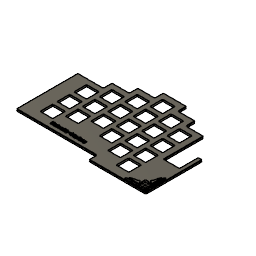
right_top (Autodesk Fusion 360 design; units mm, degrees)
part number: 2026-06-20-00-17-14-942
Autodesk Fusion 360 part; units mm, degrees
(part 1 of 2)
sketch "Sketch1" plane through (0, 0, 0) normal (0, 0, 1) x (1, 0, 0)
  line L0 (0.7819, 35.4718) -> (13.7819, 35.4718)
  line L1 (0.7819, 21.4718) -> (13.7819, 21.4718)
  line L2 (0.2819, 34.9718) -> (0.2819, 21.9718)
  line L3 (14.2819, 34.9718) -> (14.2819, 21.9718)
  arc A0 (0.7819, 35.4718) -> (0.2819, 34.9718) centre (0.7819, 34.9718) ccw
  arc A1 (14.2819, 34.9718) -> (13.7819, 35.4718) centre (13.7819, 34.9718) ccw
  arc A2 (0.2819, 21.9718) -> (0.7819, 21.4718) centre (0.7819, 21.9718) ccw
  arc A3 (13.7819, 21.4718) -> (14.2819, 21.9718) centre (13.7819, 21.9718) ccw
  line L4 (-18.2681, 25.9468) -> (-5.2681, 25.9468)
  line L5 (-18.2681, 11.9468) -> (-5.2681, 11.9468)
  line L6 (-18.7681, 25.4468) -> (-18.7681, 12.4468)
  line L7 (-4.7681, 25.4468) -> (-4.7681, 12.4468)
  arc A4 (-18.2681, 25.9468) -> (-18.7681, 25.4468) centre (-18.2681, 25.4468) ccw
  arc A5 (-4.7681, 25.4468) -> (-5.2681, 25.9468) centre (-5.2681, 25.4468) ccw
  arc A6 (-18.7681, 12.4468) -> (-18.2681, 11.9468) centre (-18.2681, 12.4468) ccw
  arc A7 (-5.2681, 11.9468) -> (-4.7681, 12.4468) centre (-5.2681, 12.4468) ccw
  line L8 (19.8319, 25.9468) -> (32.8319, 25.9468)
  line L9 (19.8319, 11.9468) -> (32.8319, 11.9468)
  line L10 (19.3319, 25.4468) -> (19.3319, 12.4468)
  line L11 (33.3319, 25.4468) -> (33.3319, 12.4468)
  arc A8 (19.8319, 25.9468) -> (19.3319, 25.4468) centre (19.8319, 25.4468) ccw
  arc A9 (33.3319, 25.4468) -> (32.8319, 25.9468) centre (32.8319, 25.4468) ccw
  arc A10 (19.3319, 12.4468) -> (19.8319, 11.9468) centre (19.8319, 12.4468) ccw
  arc A11 (32.8319, 11.9468) -> (33.3319, 12.4468) centre (32.8319, 12.4468) ccw
  line L12 (-37.3181, 16.4218) -> (-24.3181, 16.4218)
  line L13 (-37.3181, 2.4218) -> (-24.3181, 2.4218)
  line L14 (-37.8181, 15.9218) -> (-37.8181, 2.9218)
  line L15 (-23.8181, 15.9218) -> (-23.8181, 2.9218)
  arc A12 (-37.3181, 16.4218) -> (-37.8181, 15.9218) centre (-37.3181, 15.9218) ccw
  arc A13 (-23.8181, 15.9218) -> (-24.3181, 16.4218) centre (-24.3181, 15.9218) ccw
  arc A14 (-37.8181, 2.9218) -> (-37.3181, 2.4218) centre (-37.3181, 2.9218) ccw
  arc A15 (-24.3181, 2.4218) -> (-23.8181, 2.9218) centre (-24.3181, 2.9218) ccw
  line L16 (0.7819, 16.4218) -> (13.7819, 16.4218)
  line L17 (0.7819, 2.4218) -> (13.7819, 2.4218)
  line L18 (0.2819, 15.9218) -> (0.2819, 2.9218)
  line L19 (14.2819, 15.9218) -> (14.2819, 2.9218)
  arc A16 (0.7819, 16.4218) -> (0.2819, 15.9218) centre (0.7819, 15.9218) ccw
  arc A17 (14.2819, 15.9218) -> (13.7819, 16.4218) centre (13.7819, 15.9218) ccw
  arc A18 (0.2819, 2.9218) -> (0.7819, 2.4218) centre (0.7819, 2.9218) ccw
  arc A19 (13.7819, 2.4218) -> (14.2819, 2.9218) centre (13.7819, 2.9218) ccw
  line L20 (38.8819, 16.4218) -> (51.8819, 16.4218)
  line L21 (38.8819, 2.4218) -> (51.8819, 2.4218)
  line L22 (38.3819, 15.9218) -> (38.3819, 2.9218)
  line L23 (52.3819, 15.9218) -> (52.3819, 2.9218)
  arc A20 (38.8819, 16.4218) -> (38.3819, 15.9218) centre (38.8819, 15.9218) ccw
  arc A21 (52.3819, 15.9218) -> (51.8819, 16.4218) centre (51.8819, 15.9218) ccw
  arc A22 (38.3819, 2.9218) -> (38.8819, 2.4218) centre (38.8819, 2.9218) ccw
  arc A23 (51.8819, 2.4218) -> (52.3819, 2.9218) centre (51.8819, 2.9218) ccw
  line L24 (-56.3681, 6.8968) -> (-43.3681, 6.8968)
  line L25 (-56.3681, -7.1032) -> (-43.3681, -7.1032)
  line L26 (-56.8681, 6.3968) -> (-56.8681, -6.6032)
  line L27 (-42.8681, 6.3968) -> (-42.8681, -6.6032)
  arc A24 (-56.3681, 6.8968) -> (-56.8681, 6.3968) centre (-56.3681, 6.3968) ccw
  arc A25 (-42.8681, 6.3968) -> (-43.3681, 6.8968) centre (-43.3681, 6.3968) ccw
  arc A26 (-56.8681, -6.6032) -> (-56.3681, -7.1032) centre (-56.3681, -6.6032) ccw
  arc A27 (-43.3681, -7.1032) -> (-42.8681, -6.6032) centre (-43.3681, -6.6032) ccw
  line L28 (-18.2681, 6.8968) -> (-5.2681, 6.8968)
  line L29 (-18.2681, -7.1032) -> (-5.2681, -7.1032)
  line L30 (-18.7681, 6.3968) -> (-18.7681, -6.6032)
  line L31 (-4.7681, 6.3968) -> (-4.7681, -6.6032)
  arc A28 (-18.2681, 6.8968) -> (-18.7681, 6.3968) centre (-18.2681, 6.3968) ccw
  arc A29 (-4.7681, 6.3968) -> (-5.2681, 6.8968) centre (-5.2681, 6.3968) ccw
  arc A30 (-18.7681, -6.6032) -> (-18.2681, -7.1032) centre (-18.2681, -6.6032) ccw
  arc A31 (-5.2681, -7.1032) -> (-4.7681, -6.6032) centre (-5.2681, -6.6032) ccw
  line L32 (19.8319, 6.8968) -> (32.8319, 6.8968)
  line L33 (19.8319, -7.1032) -> (32.8319, -7.1032)
  line L34 (19.3319, 6.3968) -> (19.3319, -6.6032)
  line L35 (33.3319, 6.3968) -> (33.3319, -6.6032)
  arc A32 (19.8319, 6.8968) -> (19.3319, 6.3968) centre (19.8319, 6.3968) ccw
  arc A33 (33.3319, 6.3968) -> (32.8319, 6.8968) centre (32.8319, 6.3968) ccw
  arc A34 (19.3319, -6.6032) -> (19.8319, -7.1032) centre (19.8319, -6.6032) ccw
  arc A35 (32.8319, -7.1032) -> (33.3319, -6.6032) centre (32.8319, -6.6032) ccw
  line L36 (-37.3181, -2.6282) -> (-24.3181, -2.6282)
  line L37 (-37.3181, -16.6282) -> (-24.3181, -16.6282)
  line L38 (-37.8181, -3.1282) -> (-37.8181, -16.1282)
  line L39 (-23.8181, -3.1282) -> (-23.8181, -16.1282)
  arc A36 (-37.3181, -2.6282) -> (-37.8181, -3.1282) centre (-37.3181, -3.1282) ccw
  arc A37 (-23.8181, -3.1282) -> (-24.3181, -2.6282) centre (-24.3181, -3.1282) ccw
  arc A38 (-37.8181, -16.1282) -> (-37.3181, -16.6282) centre (-37.3181, -16.1282) ccw
  arc A39 (-24.3181, -16.6282) -> (-23.8181, -16.1282) centre (-24.3181, -16.1282) ccw
  line L40 (0.7819, -2.6282) -> (13.7819, -2.6282)
  line L41 (0.7819, -16.6282) -> (13.7819, -16.6282)
  line L42 (0.2819, -3.1282) -> (0.2819, -16.1282)
  line L43 (14.2819, -3.1282) -> (14.2819, -16.1282)
  arc A40 (0.7819, -2.6282) -> (0.2819, -3.1282) centre (0.7819, -3.1282) ccw
  arc A41 (14.2819, -3.1282) -> (13.7819, -2.6282) centre (13.7819, -3.1282) ccw
  arc A42 (0.2819, -16.1282) -> (0.7819, -16.6282) centre (0.7819, -16.1282) ccw
  arc A43 (13.7819, -16.6282) -> (14.2819, -16.1282) centre (13.7819, -16.1282) ccw
  line L44 (38.8819, -2.6282) -> (51.8819, -2.6282)
  line L45 (38.8819, -16.6282) -> (51.8819, -16.6282)
  line L46 (38.3819, -3.1282) -> (38.3819, -16.1282)
  line L47 (52.3819, -3.1282) -> (52.3819, -16.1282)
  arc A44 (38.8819, -2.6282) -> (38.3819, -3.1282) centre (38.8819, -3.1282) ccw
  arc A45 (52.3819, -3.1282) -> (51.8819, -2.6282) centre (51.8819, -3.1282) ccw
  arc A46 (38.3819, -16.1282) -> (38.8819, -16.6282) centre (38.8819, -16.1282) ccw
  arc A47 (51.8819, -16.6282) -> (52.3819, -16.1282) centre (51.8819, -16.1282) ccw
  line L48 (-56.3681, -12.1532) -> (-43.3681, -12.1532)
  line L49 (-56.3681, -26.1532) -> (-43.3681, -26.1532)
  line L50 (-56.8681, -12.6532) -> (-56.8681, -25.6532)
  line L51 (-42.8681, -12.6532) -> (-42.8681, -25.6532)
  arc A48 (-56.3681, -12.1532) -> (-56.8681, -12.6532) centre (-56.3681, -12.6532) ccw
  arc A49 (-42.8681, -12.6532) -> (-43.3681, -12.1532) centre (-43.3681, -12.6532) ccw
  arc A50 (-56.8681, -25.6532) -> (-56.3681, -26.1532) centre (-56.3681, -25.6532) ccw
  arc A51 (-43.3681, -26.1532) -> (-42.8681, -25.6532) centre (-43.3681, -25.6532) ccw
  line L52 (-18.2681, -12.1532) -> (-5.2681, -12.1532)
  line L53 (-18.2681, -26.1532) -> (-5.2681, -26.1532)
  line L54 (-18.7681, -12.6532) -> (-18.7681, -25.6532)
  line L55 (-4.7681, -12.6532) -> (-4.7681, -25.6532)
  arc A52 (-18.2681, -12.1532) -> (-18.7681, -12.6532) centre (-18.2681, -12.6532) ccw
  arc A53 (-4.7681, -12.6532) -> (-5.2681, -12.1532) centre (-5.2681, -12.6532) ccw
  arc A54 (-18.7681, -25.6532) -> (-18.2681, -26.1532) centre (-18.2681, -25.6532) ccw
  arc A55 (-5.2681, -26.1532) -> (-4.7681, -25.6532) centre (-5.2681, -25.6532) ccw
  line L56 (19.8319, -12.1532) -> (32.8319, -12.1532)
  line L57 (19.8319, -26.1532) -> (32.8319, -26.1532)
  line L58 (19.3319, -12.6532) -> (19.3319, -25.6532)
  line L59 (33.3319, -12.6532) -> (33.3319, -25.6532)
  arc A56 (19.8319, -12.1532) -> (19.3319, -12.6532) centre (19.8319, -12.6532) ccw
  arc A57 (33.3319, -12.6532) -> (32.8319, -12.1532) centre (32.8319, -12.6532) ccw
  arc A58 (19.3319, -25.6532) -> (19.8319, -26.1532) centre (19.8319, -25.6532) ccw
  arc A59 (32.8319, -26.1532) -> (33.3319, -25.6532) centre (32.8319, -25.6532) ccw
  line L60 (-37.3181, -21.6782) -> (-24.3181, -21.6782)
  line L61 (-37.3181, -35.6782) -> (-24.3181, -35.6782)
  line L62 (-37.8181, -22.1782) -> (-37.8181, -35.1782)
  line L63 (-23.8181, -22.1782) -> (-23.8181, -35.1782)
  arc A60 (-37.3181, -21.6782) -> (-37.8181, -22.1782) centre (-37.3181, -22.1782) ccw
  arc A61 (-23.8181, -22.1782) -> (-24.3181, -21.6782) centre (-24.3181, -22.1782) ccw
  arc A62 (-37.8181, -35.1782) -> (-37.3181, -35.6782) centre (-37.3181, -35.1782) ccw
  arc A63 (-24.3181, -35.6782) -> (-23.8181, -35.1782) centre (-24.3181, -35.1782) ccw
  line L64 (0.7819, -21.6782) -> (13.7819, -21.6782)
  line L65 (0.7819, -35.6782) -> (13.7819, -35.6782)
  line L66 (0.2819, -22.1782) -> (0.2819, -35.1782)
  line L67 (14.2819, -22.1782) -> (14.2819, -35.1782)
  arc A64 (0.7819, -21.6782) -> (0.2819, -22.1782) centre (0.7819, -22.1782) ccw
  arc A65 (14.2819, -22.1782) -> (13.7819, -21.6782) centre (13.7819, -22.1782) ccw
  arc A66 (0.2819, -35.1782) -> (0.7819, -35.6782) centre (0.7819, -35.1782) ccw
  arc A67 (13.7819, -35.6782) -> (14.2819, -35.1782) centre (13.7819, -35.1782) ccw
  line L68 (38.8819, -21.6782) -> (51.8819, -21.6782)
  line L69 (38.8819, -35.6782) -> (51.8819, -35.6782)
  line L70 (38.3819, -22.1782) -> (38.3819, -35.1782)
  line L71 (52.3819, -22.1782) -> (52.3819, -35.1782)
  arc A68 (38.8819, -21.6782) -> (38.3819, -22.1782) centre (38.8819, -22.1782) ccw
  arc A69 (52.3819, -22.1782) -> (51.8819, -21.6782) centre (51.8819, -22.1782) ccw
  arc A70 (38.3819, -35.1782) -> (38.8819, -35.6782) centre (38.8819, -35.1782) ccw
  arc A71 (51.8819, -35.6782) -> (52.3819, -35.1782) centre (51.8819, -35.1782) ccw
  line L72 (-56.3681, -31.2032) -> (-43.3681, -31.2032)
  line L73 (-56.3681, -45.2032) -> (-43.3681, -45.2032)
  line L74 (-56.8681, -31.7032) -> (-56.8681, -44.7032)
  line L75 (-42.8681, -31.7032) -> (-42.8681, -44.7032)
  arc A72 (-56.3681, -31.2032) -> (-56.8681, -31.7032) centre (-56.3681, -31.7032) ccw
  arc A73 (-42.8681, -31.7032) -> (-43.3681, -31.2032) centre (-43.3681, -31.7032) ccw
  arc A74 (-56.8681, -44.7032) -> (-56.3681, -45.2032) centre (-56.3681, -44.7032) ccw
  arc A75 (-43.3681, -45.2032) -> (-42.8681, -44.7032) centre (-43.3681, -44.7032) ccw
  line L76 (19.8319, -31.2032) -> (32.8319, -31.2032)
  line L77 (19.8319, -45.2032) -> (32.8319, -45.2032)
  line L78 (19.3319, -31.7032) -> (19.3319, -44.7032)
  line L79 (33.3319, -31.7032) -> (33.3319, -44.7032)
  arc A76 (19.8319, -31.2032) -> (19.3319, -31.7032) centre (19.8319, -31.7032) ccw
  arc A77 (33.3319, -31.7032) -> (32.8319, -31.2032) centre (32.8319, -31.7032) ccw
  arc A78 (19.3319, -44.7032) -> (19.8319, -45.2032) centre (19.8319, -44.7032) ccw
  arc A79 (32.8319, -45.2032) -> (33.3319, -44.7032) centre (32.8319, -44.7032) ccw
  line L80 (38.8819, -40.7282) -> (51.8819, -40.7282)
  line L81 (38.8819, -54.7282) -> (51.8819, -54.7282)
  line L82 (38.3819, -41.2282) -> (38.3819, -54.2282)
  line L83 (52.3819, -41.2282) -> (52.3819, -54.2282)
  arc A80 (38.8819, -40.7282) -> (38.3819, -41.2282) centre (38.8819, -41.2282) ccw
  arc A81 (52.3819, -41.2282) -> (51.8819, -40.7282) centre (51.8819, -41.2282) ccw
  arc A82 (38.3819, -54.2282) -> (38.8819, -54.7282) centre (38.8819, -54.2282) ccw
  arc A83 (51.8819, -54.7282) -> (52.3819, -54.2282) centre (51.8819, -54.2282) ccw
  line L84 (17.5099, -64.7813) -> (17.5099, -56.2276)
  line L85 (-22.2728, 20.5218) -> (-22.268, 30.0689)
  line L86 (-44.2453, 13.2468) -> (-72.9981, 13.2468)
  line L87 (56.9999, -3.4713) -> (79.0907, -3.4527)
  line L88 (-5.6619, 32.5689) -> (-5.6619, 42.2137)
  line L89 (18.2399, 30.3487) -> (37.2999, 30.3337)
  line L90 (-70.5308, -53.7443) -> (-70.4981, 10.7468)
  line L91 (20.0142, -53.7276) -> (-70.5308, -53.7443)
  line L92 (79.0907, -62.2813) -> (20.0099, -62.2513)
  line L93 (56.9799, 20.2585) -> (56.9999, -3.4713)
  line L94 (-5.6619, 42.2137) -> (20.7399, 42.2137)
  line L95 (37.2998, 20.2585) -> (56.9799, 20.2585)
  line L96 (59.4799, 22.7585) -> (59.4799, -0.9527)
  line L97 (-3.1619, 39.7137) -> (18.2399, 39.7137)
  line L98 (-70.4981, 10.7468) -> (-41.7503, 10.7468)
  line L99 (-22.268, 30.0689) -> (-3.1619, 30.0592)
  line L100 (-24.7728, 23.0218) -> (-24.7728, 32.5689)
  line L101 (20.7399, 42.2137) -> (20.7399, 32.8337)
  line L102 (39.7999, 32.8337) -> (39.7999, 22.7585)
  line L103 (81.5907, -64.7813) -> (17.5099, -64.7813)
  line L104 (18.2399, 39.7137) -> (18.2399, 30.3487)
  line L105 (-44.2453, 23.0218) -> (-24.7728, 23.0218)
  line L106 (17.5099, -56.2276) -> (-72.9981, -56.2276)
  line L107 (-72.9981, -56.2276) -> (-72.9981, 13.2468)
  line L108 (-44.2453, 23.0218) -> (-44.2453, 13.2468)
  line L109 (81.5907, -0.9527) -> (81.5907, -64.7813)
  line L110 (39.7999, 22.7585) -> (59.4799, 22.7585)
  line L111 (39.7999, 32.8337) -> (20.7399, 32.8337)
  line L112 (-3.1619, 30.0592) -> (-3.1619, 39.7137)
  line L113 (20.0099, -62.2513) -> (20.0142, -53.7276)
  line L114 (37.2999, 30.3337) -> (37.2999, 20.3074)
  line L115 (-41.7503, 10.7468) -> (-41.7453, 20.5218)
  line L116 (79.0907, -3.4527) -> (79.0907, -62.2813)
  line L117 (-24.7728, 32.5689) -> (-5.6619, 32.5689)
  line L118 (-41.7453, 20.5218) -> (-22.2728, 20.5218)
  line L119 (37.2999, 20.3074) -> (37.2998, 20.2585)
  line L120 (81.5907, -0.9527) -> (59.4799, -0.9527)
  line L121 (59.4799, -0.9527) -> (77, -0.9527)
  line L122 (77, -0.9527) -> (77, -22.2268)
  line L123 (77, -22.2268) -> (59.4799, -22.2268)
  line L124 (59.4799, -22.2268) -> (59.4799, -0.9527)
  point P0 (11.0021, -13.517)
  dimension "d1" = 2.5
  dimension "d2" = 2.5
  dimension "d3" = 2.5
  dimension "d4" = 2.5
  dimension "d5" = 2.5
  dimension "d6" = 2.5
  dimension "d7" = 2.5
  dimension "d8" = 2.5
  dimension "d9" = 2.5
  dimension "d10" = 2.5
  dimension "d11" = 2.5
  dimension "d12" = 2.5
  dimension "d13" = 2.5
  dimension "d14" = 2.5
  dimension "d15" = 2.5
  dimension "d16" = 2.5
  dimension "d17" = 2.5
  dimension "d18" = 2.5
  dimension "d19" = 2.5
  dimension "d20" = 16.13
  dimension "d21" = 6.35
  dimension "d22" = 17.5201
  constraint parallel L90 L115
  constraint parallel L98 L118
  constraint parallel L85 L90
  constraint perpendicular L85 L99
  constraint vertical L112
  constraint perpendicular L97 L112
  constraint perpendicular L97 L104
  constraint parallel L104 L114
  constraint perpendicular L89 L119
  constraint perpendicular L95 L104
  constraint perpendicular L87 L93
  constraint perpendicular L95 L116
  constraint perpendicular L92 L113
  constraint horizontal L86
  constraint vertical L108
  constraint horizontal L105
  constraint perpendicular L100 L105
  constraint perpendicular L112 L117
  constraint perpendicular L88 L117
  constraint coincident L88.start L117
  constraint horizontal L94
  constraint coincident L88.end L94
  constraint vertical L101
  constraint perpendicular L101 L111
  constraint coincident L111.end L101
  constraint vertical L102
  constraint coincident L111.start L102
  constraint horizontal L110
  constraint perpendicular L96 L110
  constraint horizontal L120
  constraint perpendicular L109 L120
  constraint perpendicular L103 L116
  constraint coincident L103.start L109
  constraint perpendicular L84 L103
  constraint coincident L103.end L84
  constraint horizontal L106
  constraint coincident L84.end L106
  constraint perpendicular L106 L107
  constraint coincident L86.end L107
  constraint coincident L107.start L106
  constraint horizontal L121
  constraint vertical L122
  constraint horizontal L123
  constraint vertical L124
  measures "d1" vertical distance of L90.end L86.end
  measures "d2" horizontal distance of L115.end L105.start
  measures "d3" vertical distance of L86.start L98.end
  measures "d4" vertical distance of L115.end L105.start
  measures "d5" horizontal distance of L85.start L100.start
  measures "d6" vertical distance of L85.end L100.end
  measures "d7" horizontal distance of L97.start L88.end
  measures "d8" vertical distance of L97.start L88.end
  measures "d9" horizontal distance of L94.end L97.end
  measures "d10" vertical distance of L102.start L89.end
  measures "d11" horizontal distance of L102.start L89.end
  measures "d12" vertical distance of L93.start L96.start
  measures "d13" horizontal distance of L93.start L96.start
  measures "d14" vertical distance of L96.end L87.end
  measures "d15" horizontal distance of L109.start L87.end
  measures "d16" vertical distance of L92.start L103.start
  measures "d17" horizontal distance of L84.start L92.end
  measures "d18" vertical distance of L84.end L91.start
  measures "d19" horizontal distance of L90.end L86.end
  measures "d20" distance of L26 L107
  measures "d21" distance of L24 L86
  measures "d22" distance of L122 L124
extrude "Extrude1" add sketch "Sketch1" along normal blind 2 contours L84 L85 L86 L87 L88 L89 L90 L91 L92 L93 L94 L95 L96 L97 L98 L99 L100 L101 L102 L103 L104 L105 L106 L107 L108 L109 L110 L111 L112 L113 L114 L115 L116 L117 L118 L119 L120 L122 L124 | L85 L87 L89 L90 L91 L92 L93 L95 L97 L98 L99 L104 L112 L113 L114 L115 L116 L118 L119 L122 L123 L124
fillet "Fillet1" radius 1 17 edges at (81.5907, -64.7813, 1) (17.5099, -64.7813, 1) (81.5907, -0.9527, 1) (59.4799, 22.7585, 1) (39.7999, 32.8337, 1) (20.7399, 42.2137, 1) (-72.9981, -56.2276, 1) (17.5099, -56.2276, 1) (-72.9981, 13.2468, 1) (-44.2453, 23.0218, 1) (-24.7728, 32.5689, 1) (-5.6619, 42.2137, 1) (-5.6619, 32.5689, 1) (-24.7728, 23.0218, 1) (-44.2453, 13.2468, 1) (20.7399, 32.8337, 1) (39.7999, 22.7585, 1)
fillet "Fillet2" radius 0.3 37 edges at (59.4799, -0.2342, 2) (59.187, 22.4656, 2) (49.6399, 22.7585, 2) (40.0928, 23.0514, 2) (39.7999, 27.7961, 2) (39.507, 32.5408, 2) (30.2699, 32.8337, 2) (21.0328, 33.1266, 2) (20.7399, 37.5237, 2) (20.447, 41.9208, 2) (7.539, 42.2137, 2) (-5.3691, 41.9208, 2) (-5.6619, 37.3913, 2) (-5.9548, 32.8618, 2) (-15.2174, 32.5689, 2) (-24.4799, 32.276, 2) (-24.7728, 27.7953, 2) (-25.0657, 23.3146, 2) (-34.5091, 23.0218, 2) (-43.9525, 22.7289, 2) (-44.2453, 18.1343, 2) (-44.5382, 13.5397, 2) (-58.6217, 13.2468, 2) (-72.7052, 12.9539, 2) (-72.9981, -21.4904, 2) (-72.7052, -55.9347, 2) (-27.7441, -56.2276, 2) (17.217, -56.5205, 2) (17.5099, -60.5045, 2) (17.8028, -64.4884, 2) (49.5503, -64.7813, 2) (81.2978, -64.4884, 2) (81.5907, -32.867, 2) (81.2978, -1.2456, 2) (78.7954, -0.9527, 2) (68.2399, -22.2268, 2) (77, -11.5898, 2)
sketch "Sketch2" plane through (0, 0, 2) normal (0, 0, 1) x (-1, 0, 0)
  arc A0 (-38.8819, 21.6782) -> (-38.3819, 22.1782) centre (-38.8819, 22.1782) ccw
  line L0 (-38.8819, 21.6782) -> (-51.8819, 21.6782)
  arc A1 (-52.3819, 22.1782) -> (-51.8819, 21.6782) centre (-51.8819, 22.1782) ccw
  line L1 (-52.3819, 22.1782) -> (-52.3819, 35.1782)
  arc A2 (-51.8819, 35.6782) -> (-52.3819, 35.1782) centre (-51.8819, 35.1782) ccw
  line L2 (-51.8819, 35.6782) -> (-38.8819, 35.6782)
  arc A3 (-38.3819, 35.1782) -> (-38.8819, 35.6782) centre (-38.8819, 35.1782) ccw
  line L3 (-38.3819, 35.1782) -> (-38.3819, 22.1782)
  arc A4 (37.3181, 21.6782) -> (37.8181, 22.1782) centre (37.3181, 22.1782) ccw
  line L4 (37.3181, 21.6782) -> (24.3181, 21.6782)
  arc A5 (23.8181, 22.1782) -> (24.3181, 21.6782) centre (24.3181, 22.1782) ccw
  line L5 (23.8181, 22.1782) -> (23.8181, 35.1782)
  arc A6 (24.3181, 35.6782) -> (23.8181, 35.1782) centre (24.3181, 35.1782) ccw
  line L6 (24.3181, 35.6782) -> (37.3181, 35.6782)
  arc A7 (37.8181, 35.1782) -> (37.3181, 35.6782) centre (37.3181, 35.1782) ccw
  line L7 (37.8181, 35.1782) -> (37.8181, 22.1782)
  arc A8 (-0.7819, -35.4718) -> (-0.2819, -34.9718) centre (-0.7819, -34.9718) ccw
  line L8 (-0.7819, -35.4718) -> (-13.7819, -35.4718)
  arc A9 (-14.2819, -34.9718) -> (-13.7819, -35.4718) centre (-13.7819, -34.9718) ccw
  line L9 (-14.2819, -34.9718) -> (-14.2819, -21.9718)
  arc A10 (-13.7819, -21.4718) -> (-14.2819, -21.9718) centre (-13.7819, -21.9718) ccw
  line L10 (-13.7819, -21.4718) -> (-0.7819, -21.4718)
  arc A11 (-0.2819, -21.9718) -> (-0.7819, -21.4718) centre (-0.7819, -21.9718) ccw
  line L11 (-0.2819, -21.9718) -> (-0.2819, -34.9718)
  arc A12 (-0.7819, 21.6782) -> (-0.2819, 22.1782) centre (-0.7819, 22.1782) ccw
  line L12 (-0.7819, 21.6782) -> (-13.7819, 21.6782)
  arc A13 (-14.2819, 22.1782) -> (-13.7819, 21.6782) centre (-13.7819, 22.1782) ccw
  line L13 (-14.2819, 22.1782) -> (-14.2819, 35.1782)
  arc A14 (-13.7819, 35.6782) -> (-14.2819, 35.1782) centre (-13.7819, 35.1782) ccw
  line L14 (-13.7819, 35.6782) -> (-0.7819, 35.6782)
  arc A15 (-0.2819, 35.1782) -> (-0.7819, 35.6782) centre (-0.7819, 35.1782) ccw
  line L15 (-0.2819, 35.1782) -> (-0.2819, 22.1782)
  arc A16 (18.2681, -25.9468) -> (18.7681, -25.4468) centre (18.2681, -25.4468) ccw
  line L16 (18.2681, -25.9468) -> (5.2681, -25.9468)
  arc A17 (4.7681, -25.4468) -> (5.2681, -25.9468) centre (5.2681, -25.4468) ccw
  line L17 (4.7681, -25.4468) -> (4.7681, -12.4468)
  arc A18 (5.2681, -11.9468) -> (4.7681, -12.4468) centre (5.2681, -12.4468) ccw
  line L18 (5.2681, -11.9468) -> (18.2681, -11.9468)
  arc A19 (18.7681, -12.4468) -> (18.2681, -11.9468) centre (18.2681, -12.4468) ccw
  line L19 (18.7681, -12.4468) -> (18.7681, -25.4468)
  arc A20 (-0.7819, 2.6282) -> (-0.2819, 3.1282) centre (-0.7819, 3.1282) ccw
  line L20 (-0.7819, 2.6282) -> (-13.7819, 2.6282)
  arc A21 (-14.2819, 3.1282) -> (-13.7819, 2.6282) centre (-13.7819, 3.1282) ccw
  line L21 (-14.2819, 3.1282) -> (-14.2819, 16.1282)
  arc A22 (-13.7819, 16.6282) -> (-14.2819, 16.1282) centre (-13.7819, 16.1282) ccw
  line L22 (-13.7819, 16.6282) -> (-0.7819, 16.6282)
  arc A23 (-0.2819, 16.1282) -> (-0.7819, 16.6282) centre (-0.7819, 16.1282) ccw
  line L23 (-0.2819, 16.1282) -> (-0.2819, 3.1282)
  arc A24 (-19.8319, -6.8968) -> (-19.3319, -6.3968) centre (-19.8319, -6.3968) ccw
  line L24 (-19.8319, -6.8968) -> (-32.8319, -6.8968)
  arc A25 (-33.3319, -6.3968) -> (-32.8319, -6.8968) centre (-32.8319, -6.3968) ccw
  line L25 (-33.3319, -6.3968) -> (-33.3319, 6.6032)
  arc A26 (-32.8319, 7.1032) -> (-33.3319, 6.6032) centre (-32.8319, 6.6032) ccw
  line L26 (-32.8319, 7.1032) -> (-19.8319, 7.1032)
  arc A27 (-19.3319, 6.6032) -> (-19.8319, 7.1032) centre (-19.8319, 6.6032) ccw
  line L27 (-19.3319, 6.6032) -> (-19.3319, -6.3968)
  arc A28 (56.3681, 31.2032) -> (56.8681, 31.7032) centre (56.3681, 31.7032) ccw
  line L28 (56.3681, 31.2032) -> (43.3681, 31.2032)
  arc A29 (42.8681, 31.7032) -> (43.3681, 31.2032) centre (43.3681, 31.7032) ccw
  line L29 (42.8681, 31.7032) -> (42.8681, 44.7032)
  arc A30 (43.3681, 45.2032) -> (42.8681, 44.7032) centre (43.3681, 44.7032) ccw
  line L30 (43.3681, 45.2032) -> (56.3681, 45.2032)
  arc A31 (56.8681, 44.7032) -> (56.3681, 45.2032) centre (56.3681, 44.7032) ccw
  line L31 (56.8681, 44.7032) -> (56.8681, 31.7032)
  arc A32 (37.3181, -16.4218) -> (37.8181, -15.9218) centre (37.3181, -15.9218) ccw
  line L32 (37.3181, -16.4218) -> (24.3181, -16.4218)
  arc A33 (23.8181, -15.9218) -> (24.3181, -16.4218) centre (24.3181, -15.9218) ccw
  line L33 (23.8181, -15.9218) -> (23.8181, -2.9218)
  arc A34 (24.3181, -2.4218) -> (23.8181, -2.9218) centre (24.3181, -2.9218) ccw
  line L34 (24.3181, -2.4218) -> (37.3181, -2.4218)
  arc A35 (37.8181, -2.9218) -> (37.3181, -2.4218) centre (37.3181, -2.9218) ccw
  line L35 (37.8181, -2.9218) -> (37.8181, -15.9218)
  arc A36 (-19.8319, 12.1532) -> (-19.3319, 12.6532) centre (-19.8319, 12.6532) ccw
  line L36 (-19.8319, 12.1532) -> (-32.8319, 12.1532)
  arc A37 (-33.3319, 12.6532) -> (-32.8319, 12.1532) centre (-32.8319, 12.6532) ccw
  line L37 (-33.3319, 12.6532) -> (-33.3319, 25.6532)
  arc A38 (-32.8319, 26.1532) -> (-33.3319, 25.6532) centre (-32.8319, 25.6532) ccw
  line L38 (-32.8319, 26.1532) -> (-19.8319, 26.1532)
  arc A39 (-19.3319, 25.6532) -> (-19.8319, 26.1532) centre (-19.8319, 25.6532) ccw
  line L39 (-19.3319, 25.6532) -> (-19.3319, 12.6532)
  arc A40 (-19.8319, -25.9468) -> (-19.3319, -25.4468) centre (-19.8319, -25.4468) ccw
  line L40 (-19.8319, -25.9468) -> (-32.8319, -25.9468)
  arc A41 (-33.3319, -25.4468) -> (-32.8319, -25.9468) centre (-32.8319, -25.4468) ccw
  line L41 (-33.3319, -25.4468) -> (-33.3319, -12.4468)
  arc A42 (-32.8319, -11.9468) -> (-33.3319, -12.4468) centre (-32.8319, -12.4468) ccw
  line L42 (-32.8319, -11.9468) -> (-19.8319, -11.9468)
  arc A43 (-19.3319, -12.4468) -> (-19.8319, -11.9468) centre (-19.8319, -12.4468) ccw
  line L43 (-19.3319, -12.4468) -> (-19.3319, -25.4468)
  arc A44 (-38.8819, -16.4218) -> (-38.3819, -15.9218) centre (-38.8819, -15.9218) ccw
  line L44 (-38.8819, -16.4218) -> (-51.8819, -16.4218)
  arc A45 (-52.3819, -15.9218) -> (-51.8819, -16.4218) centre (-51.8819, -15.9218) ccw
  line L45 (-52.3819, -15.9218) -> (-52.3819, -2.9218)
  arc A46 (-51.8819, -2.4218) -> (-52.3819, -2.9218) centre (-51.8819, -2.9218) ccw
  line L46 (-51.8819, -2.4218) -> (-38.8819, -2.4218)
  arc A47 (-38.3819, -2.9218) -> (-38.8819, -2.4218) centre (-38.8819, -2.9218) ccw
  line L47 (-38.3819, -2.9218) -> (-38.3819, -15.9218)
  arc A48 (-38.8819, 40.7282) -> (-38.3819, 41.2282) centre (-38.8819, 41.2282) ccw
  line L48 (-38.8819, 40.7282) -> (-51.8819, 40.7282)
  arc A49 (-52.3819, 41.2282) -> (-51.8819, 40.7282) centre (-51.8819, 41.2282) ccw
  line L49 (-52.3819, 41.2282) -> (-52.3819, 54.2282)
  arc A50 (-51.8819, 54.7282) -> (-52.3819, 54.2282) centre (-51.8819, 54.2282) ccw
  line L50 (-51.8819, 54.7282) -> (-38.8819, 54.7282)
  arc A51 (-38.3819, 54.2282) -> (-38.8819, 54.7282) centre (-38.8819, 54.2282) ccw
  line L51 (-38.3819, 54.2282) -> (-38.3819, 41.2282)
  arc A52 (37.3181, 2.6282) -> (37.8181, 3.1282) centre (37.3181, 3.1282) ccw
  line L52 (37.3181, 2.6282) -> (24.3181, 2.6282)
  arc A53 (23.8181, 3.1282) -> (24.3181, 2.6282) centre (24.3181, 3.1282) ccw
  line L53 (23.8181, 3.1282) -> (23.8181, 16.1282)
  arc A54 (24.3181, 16.6282) -> (23.8181, 16.1282) centre (24.3181, 16.1282) ccw
  line L54 (24.3181, 16.6282) -> (37.3181, 16.6282)
  arc A55 (37.8181, 16.1282) -> (37.3181, 16.6282) centre (37.3181, 16.1282) ccw
  line L55 (37.8181, 16.1282) -> (37.8181, 3.1282)
  arc A56 (-19.8319, 31.2032) -> (-19.3319, 31.7032) centre (-19.8319, 31.7032) ccw
  line L56 (-19.8319, 31.2032) -> (-32.8319, 31.2032)
  arc A57 (-33.3319, 31.7032) -> (-32.8319, 31.2032) centre (-32.8319, 31.7032) ccw
  line L57 (-33.3319, 31.7032) -> (-33.3319, 44.7032)
  arc A58 (-32.8319, 45.2032) -> (-33.3319, 44.7032) centre (-32.8319, 44.7032) ccw
  line L58 (-32.8319, 45.2032) -> (-19.8319, 45.2032)
  arc A59 (-19.3319, 44.7032) -> (-19.8319, 45.2032) centre (-19.8319, 44.7032) ccw
  line L59 (-19.3319, 44.7032) -> (-19.3319, 31.7032)
  arc A60 (-38.8819, 2.6282) -> (-38.3819, 3.1282) centre (-38.8819, 3.1282) ccw
  line L60 (-38.8819, 2.6282) -> (-51.8819, 2.6282)
  arc A61 (-52.3819, 3.1282) -> (-51.8819, 2.6282) centre (-51.8819, 3.1282) ccw
  line L61 (-52.3819, 3.1282) -> (-52.3819, 16.1282)
  arc A62 (-51.8819, 16.6282) -> (-52.3819, 16.1282) centre (-51.8819, 16.1282) ccw
  line L62 (-51.8819, 16.6282) -> (-38.8819, 16.6282)
  arc A63 (-38.3819, 16.1282) -> (-38.8819, 16.6282) centre (-38.8819, 16.1282) ccw
  line L63 (-38.3819, 16.1282) -> (-38.3819, 3.1282)
  arc A64 (18.2681, -6.8968) -> (18.7681, -6.3968) centre (18.2681, -6.3968) ccw
  line L64 (18.2681, -6.8968) -> (5.2681, -6.8968)
  arc A65 (4.7681, -6.3968) -> (5.2681, -6.8968) centre (5.2681, -6.3968) ccw
  line L65 (4.7681, -6.3968) -> (4.7681, 6.6032)
  arc A66 (5.2681, 7.1032) -> (4.7681, 6.6032) centre (5.2681, 6.6032) ccw
  line L66 (5.2681, 7.1032) -> (18.2681, 7.1032)
  arc A67 (18.7681, 6.6032) -> (18.2681, 7.1032) centre (18.2681, 6.6032) ccw
  line L67 (18.7681, 6.6032) -> (18.7681, -6.3968)
  arc A68 (56.3681, -6.8968) -> (56.8681, -6.3968) centre (56.3681, -6.3968) ccw
  line L68 (56.3681, -6.8968) -> (43.3681, -6.8968)
  arc A69 (42.8681, -6.3968) -> (43.3681, -6.8968) centre (43.3681, -6.3968) ccw
  line L69 (42.8681, -6.3968) -> (42.8681, 6.6032)
  arc A70 (43.3681, 7.1032) -> (42.8681, 6.6032) centre (43.3681, 6.6032) ccw
  line L70 (43.3681, 7.1032) -> (56.3681, 7.1032)
  arc A71 (56.8681, 6.6032) -> (56.3681, 7.1032) centre (56.3681, 6.6032) ccw
  line L71 (56.8681, 6.6032) -> (56.8681, -6.3968)
  arc A72 (18.2681, 12.1532) -> (18.7681, 12.6532) centre (18.2681, 12.6532) ccw
  line L72 (18.2681, 12.1532) -> (5.2681, 12.1532)
  arc A73 (4.7681, 12.6532) -> (5.2681, 12.1532) centre (5.2681, 12.6532) ccw
  line L73 (4.7681, 12.6532) -> (4.7681, 25.6532)
  arc A74 (5.2681, 26.1532) -> (4.7681, 25.6532) centre (5.2681, 25.6532) ccw
  line L74 (5.2681, 26.1532) -> (18.2681, 26.1532)
  arc A75 (18.7681, 25.6532) -> (18.2681, 26.1532) centre (18.2681, 25.6532) ccw
  line L75 (18.7681, 25.6532) -> (18.7681, 12.6532)
  arc A76 (-0.7819, -16.4218) -> (-0.2819, -15.9218) centre (-0.7819, -15.9218) ccw
  line L76 (-0.7819, -16.4218) -> (-13.7819, -16.4218)
  arc A77 (-14.2819, -15.9218) -> (-13.7819, -16.4218) centre (-13.7819, -15.9218) ccw
  line L77 (-14.2819, -15.9218) -> (-14.2819, -2.9218)
  arc A78 (-13.7819, -2.4218) -> (-14.2819, -2.9218) centre (-13.7819, -2.9218) ccw
  line L78 (-13.7819, -2.4218) -> (-0.7819, -2.4218)
  arc A79 (-0.2819, -2.9218) -> (-0.7819, -2.4218) centre (-0.7819, -2.9218) ccw
  line L79 (-0.2819, -2.9218) -> (-0.2819, -15.9218)
  arc A80 (56.3681, 12.1532) -> (56.8681, 12.6532) centre (56.3681, 12.6532) ccw
  line L80 (56.3681, 12.1532) -> (43.3681, 12.1532)
  arc A81 (42.8681, 12.6532) -> (43.3681, 12.1532) centre (43.3681, 12.6532) ccw
  line L81 (42.8681, 12.6532) -> (42.8681, 25.6532)
  arc A82 (43.3681, 26.1532) -> (42.8681, 25.6532) centre (43.3681, 25.6532) ccw
  line L82 (43.3681, 26.1532) -> (56.3681, 26.1532)
  arc A83 (56.8681, 25.6532) -> (56.3681, 26.1532) centre (56.3681, 25.6532) ccw
  line L83 (56.8681, 25.6532) -> (56.8681, 12.6532)
  line L84 (-59.1799, 22.5268) -> (-59.1799, -21.7585)
  arc A84 (-59.1799, -21.7585) -> (-58.4799, -22.4585) centre (-58.4799, -21.7585) ccw
  line L85 (-58.4799, -22.4585) -> (-40.7999, -22.4585)
  arc A85 (-39.4999, -23.7585) -> (-40.7999, -22.4585) centre (-40.7999, -23.7585) ccw
  line L86 (-39.4999, -23.7585) -> (-39.4999, -31.8337)
  arc A86 (-39.4999, -31.8337) -> (-38.7999, -32.5337) centre (-38.7999, -31.8337) ccw
  line L87 (-38.7999, -32.5337) -> (-21.7399, -32.5337)
  arc A87 (-20.4399, -33.8337) -> (-21.7399, -32.5337) centre (-21.7399, -33.8337) ccw
  line L88 (-20.4399, -33.8337) -> (-20.4399, -41.2137)
  arc A88 (-20.4399, -41.2137) -> (-19.7399, -41.9137) centre (-19.7399, -41.2137) ccw
  line L89 (-19.7399, -41.9137) -> (4.6619, -41.9137)
  arc A89 (4.6619, -41.9137) -> (5.3619, -41.2137) centre (4.6619, -41.2137) ccw
  line L90 (5.3619, -41.2137) -> (5.3619, -33.5689)
  arc A90 (6.6619, -32.2689) -> (5.3619, -33.5689) centre (6.6619, -33.5689) ccw
  line L91 (6.6619, -32.2689) -> (23.7728, -32.2689)
  arc A91 (23.7728, -32.2689) -> (24.4728, -31.5689) centre (23.7728, -31.5689) ccw
  line L92 (24.4728, -31.5689) -> (24.4728, -24.0218)
  arc A92 (25.7728, -22.7218) -> (24.4728, -24.0218) centre (25.7728, -24.0218) ccw
  line L93 (25.7728, -22.7218) -> (43.2453, -22.7218)
  arc A93 (43.2453, -22.7218) -> (43.9453, -22.0218) centre (43.2453, -22.0218) ccw
  line L94 (43.9453, -22.0218) -> (43.9453, -14.2468)
  arc A94 (45.2453, -12.9468) -> (43.9453, -14.2468) centre (45.2453, -14.2468) ccw
  line L95 (45.2453, -12.9468) -> (71.9981, -12.9468)
  arc A95 (71.9981, -12.9468) -> (72.6981, -12.2468) centre (71.9981, -12.2468) ccw
  line L96 (72.6981, -12.2468) -> (72.6981, 55.2276)
  arc A96 (72.6981, 55.2276) -> (71.9981, 55.9276) centre (71.9981, 55.2276) ccw
  line L97 (71.9981, 55.9276) -> (-16.5099, 55.9276)
  arc A97 (-17.8099, 57.2276) -> (-16.5099, 55.9276) centre (-16.5099, 57.2276) ccw
  line L98 (-17.8099, 57.2276) -> (-17.8099, 63.7813)
  arc A98 (-17.8099, 63.7813) -> (-18.5099, 64.4813) centre (-18.5099, 63.7813) ccw
  line L99 (-18.5099, 64.4813) -> (-80.5907, 64.4813)
  arc A99 (-80.5907, 64.4813) -> (-81.2907, 63.7813) centre (-80.5907, 63.7813) ccw
  line L100 (-81.2907, 63.7813) -> (-81.2907, 1.9527)
  arc A100 (-81.2907, 1.9527) -> (-80.5907, 1.2527) centre (-80.5907, 1.9527) ccw
  line L101 (-80.5907, 1.2527) -> (-77.3, 1.2527)
  line L102 (-77.3, 1.2527) -> (-77.3, 22.5268)
  line L103 (-77.3, 22.5268) -> (-59.1799, 22.5268)
  line L104 (-78.5, 40.3) -> (-79.9, 40.3)
  line L105 (-79.9, 40.3) -> (-79.9, 57.9)
  line L106 (-79.9, 57.9) -> (-77.05, 57.9)
  line L107 (-77.05, 57.9) -> (-77.05, 59.25)
  line L108 (-77.05, 59.25) -> (-79.9, 59.25)
  line L109 (-79.9, 59.25) -> (-79.9, 63.65)
  line L110 (-79.9, 63.65) -> (-75.5, 63.65)
  line L111 (-75.5, 63.65) -> (-75.5, 60.7)
  line L112 (-75.5, 60.7) -> (-74.2, 60.7)
  line L113 (-74.2, 60.7) -> (-74.2, 63.65)
  line L114 (-74.2, 63.65) -> (-56.6, 63.65)
  line L115 (-56.6, 63.65) -> (-56.6, 62)
  line L116 (-56.6, 62) -> (-72.4, 62)
  line L117 (-72.4, 62) -> (-72.4, 60.7)
  line L118 (-72.4, 60.7) -> (-58.5, 60.7)
  line L119 (-71.3, 55) -> (-72.5, 55)
  line L120 (-72.5, 55) -> (-72.5, 56.2)
  line L121 (-72.5, 56.2) -> (-71.3, 56.2)
  line L122 (-71.3, 56.2) -> (-71.3, 55)
  line L123 (-74.2, 57.9) -> (-75.5157, 57.9)
  line L124 (-75.5157, 57.9) -> (-75.5157, 59.2608)
  line L125 (-75.5157, 59.2608) -> (-74.2, 59.2608)
  line L126 (-74.2, 59.2608) -> (-74.2, 57.9)
  line L127 (-77.05, 60.7171) -> (-78.5, 60.7171)
  line L128 (-78.5, 60.7171) -> (-78.5, 62.2)
  line L129 (-78.5, 62.2) -> (-77.05, 62.2)
  line L130 (-77.05, 62.2) -> (-77.05, 60.7171)
  line L131 (-78.5, 40.3) -> (-78.5, 56.0876)
  line L132 (-78.5, 56.0876) -> (-77.0548, 56.0876)
  line L133 (-77.0548, 56.0876) -> (-77.0548, 41.9263)
  line L134 (-72.4807, 57.9) -> (-69.7, 57.9)
  line L135 (-69.7, 57.9) -> (-69.7, 53.3)
  line L136 (-69.7, 53.3) -> (-74.2, 53.3)
  line L137 (-74.2, 53.3) -> (-74.2, 56.0978)
  line L138 (-74.2, 56.0978) -> (-75.5, 56.0978)
  line L139 (-75.5, 56.0978) -> (-75.5, 53)
  line L140 (-72.4807, 57.9) -> (-72.4807, 59.1825)
  line L141 (-72.4807, 59.1825) -> (-68.9937, 59.1825)
  spline S0 degree 5 poles (-77.0548, 41.9263) (-77.042, 41.9348) (-77.0158, 41.9536) (-76.9746, 41.9868) (-76.9163, 42.0413) (-76.8375, 42.1264) (-76.7533, 42.2283) (-76.664, 42.3464) (-76.5706, 42.4797) (-76.4745, 42.6271) (-76.377, 42.7869) (-76.2799, 42.9574) (-76.1845, 43.1368) (-76.0924, 43.3234) (-76.0045, 43.5159) (-75.9213, 43.713) (-75.8431, 43.9138) (-75.7694, 44.1179) (-75.6999, 44.3248) (-75.634, 44.5344) (-75.5708, 44.7465) (-75.5101, 44.9612) (-75.4512, 45.1783) (-75.3942, 45.3977) (-75.3393, 45.6193) (-75.2868, 45.8426) (-75.2371, 46.0673) (-75.1906, 46.2926) (-75.1478, 46.5178) (-75.1088, 46.7416) (-75.0736, 46.9629) (-75.0417, 47.1799) (-75.0127, 47.391) (-74.9857, 47.5941) (-74.9599, 47.7873) (-74.9348, 47.9691) (-74.91, 48.1379) (-74.8856, 48.2927) (-74.8621, 48.4329) (-74.8405, 48.5587) (-74.8214, 48.6709) (-74.8049, 48.7712) (-74.7898, 48.8621) (-74.773, 48.9474) (-74.7503, 49.0314) (-74.7174, 49.1183) (-74.6709, 49.2111) (-74.6095, 49.311) (-74.534, 49.4175) (-74.4466, 49.529) (-74.3503, 49.6435) (-74.2483, 49.7592) (-74.1434, 49.8754) (-74.0379, 49.9924) (-73.9336, 50.1108) (-73.8318, 50.2312) (-73.734, 50.3537) (-73.6412, 50.4774) (-73.5547, 50.5999) (-73.476, 50.7172) (-73.4063, 50.8255) (-73.3469, 50.9211) (-73.2986, 51.0022) (-73.2623, 51.069) (-73.2385, 51.1244) (-73.2281, 51.1723) (-73.2332, 51.2167) (-73.2568, 51.2606) (-73.3019, 51.3058) (-73.3693, 51.353) (-73.4569, 51.4009) (-73.5605, 51.448) (-73.6751, 51.4924) (-73.7955, 51.5333) (-73.9181, 51.5712) (-74.0404, 51.6082) (-74.1608, 51.6467) (-74.2782, 51.6893) (-74.3919, 51.7381) (-74.5013, 51.7939) (-74.6059, 51.8566) (-74.7051, 51.925) (-74.7988, 51.9974) (-74.887, 52.0719) (-74.9704, 52.1461) (-75.0495, 52.2181) (-75.1249, 52.2868) (-75.1966, 52.3524) (-75.2638, 52.417) (-75.3249, 52.4843) (-75.3783, 52.5575) (-75.4225, 52.6381) (-75.457, 52.7235) (-75.4821, 52.8077) (-75.4984, 52.8833) (-75.5069, 52.9435) (-75.5078, 52.9763) (-75.5051, 52.9917) (-75.502, 52.9979) (-75.5, 53) knots 0 0 0 0 0 0 0.01052632 0.02105263 0.03157895 0.04210526 0.05263158 0.06315789 0.07368421 0.08421053 0.09473684 0.10526316 0.11578947 0.12631579 0.13684211 0.14736842 0.15789474 0.16842105 0.17894737 0.18947368 0.2 0.21052632 0.22105263 0.23157895 0.24210526 0.25263158 0.26315789 0.27368421 0.28421053 0.29473684 0.30526316 0.31578947 0.32631579 0.33684211 0.34736842 0.35789474 0.36842105 0.37894737 0.38947368 0.4 0.41052632 0.42105263 0.43157895 0.44210526 0.45263158 0.46315789 0.47368421 0.48421053 0.49473684 0.50526316 0.51578947 0.52631579 0.53684211 0.54736842 0.55789474 0.56842105 0.57894737 0.58947368 0.6 0.61052632 0.62105263 0.63157895 0.64210526 0.65263158 0.66315789 0.67368421 0.68421053 0.69473684 0.70526316 0.71578947 0.72631579 0.73684211 0.74736842 0.75789474 0.76842105 0.77894737 0.78947368 0.8 0.81052632 0.82105263 0.83157895 0.84210526 0.85263158 0.86315789 0.87368421 0.88421053 0.89473684 0.90526316 0.91578947 0.92631579 0.93684211 0.94736842 0.95789474 0.96842105 0.97894737 0.98947368 1 1 1 1 1 1
  spline S1 degree 5 poles (-68.9937, 59.1825) (-68.9782, 59.1714) (-68.9475, 59.1496) (-68.9018, 59.1187) (-68.8418, 59.0809) (-68.7682, 59.0385) (-68.6965, 58.9988) (-68.6276, 58.9575) (-68.5627, 58.9072) (-68.5032, 58.8401) (-68.4499, 58.75) (-68.4028, 58.6344) (-68.36, 58.4969) (-68.3192, 58.3449) (-68.2775, 58.1878) (-68.2323, 58.0348) (-68.1819, 57.8935) (-68.126, 57.7676) (-68.0658, 57.6559) (-68.0035, 57.5546) (-67.9408, 57.4597) (-67.8788, 57.3681) (-67.8166, 57.2803) (-67.7513, 57.2008) (-67.6795, 57.1359) (-67.5978, 57.0918) (-67.5043, 57.0731) (-67.3994, 57.0802) (-67.2855, 57.1112) (-67.1662, 57.1621) (-67.0459, 57.228) (-66.9295, 57.3039) (-66.8214, 57.3855) (-66.7251, 57.469) (-66.6423, 57.5514) (-66.5721, 57.6306) (-66.5101, 57.7055) (-66.4488, 57.776) (-66.3798, 57.8428) (-66.2958, 57.9066) (-66.1928, 57.9679) (-66.0718, 58.0267) (-65.9371, 58.0827) (-65.7948, 58.1354) (-65.6509, 58.1843) (-65.51, 58.229) (-65.3733, 58.2695) (-65.2389, 58.3062) (-65.1027, 58.3397) (-64.96, 58.3706) (-64.8063, 58.3998) (-64.6383, 58.4278) (-64.4553, 58.455) (-64.2586, 58.4818) (-64.0509, 58.5082) (-63.8356, 58.5344) (-63.6167, 58.5607) (-63.3979, 58.5873) (-63.1824, 58.6148) (-62.9719, 58.6439) (-62.7668, 58.6755) (-62.5667, 58.7106) (-62.3702, 58.7503) (-62.176, 58.7953) (-61.9822, 58.846) (-61.7875, 58.9026) (-61.591, 58.9644) (-61.3926, 59.0303) (-61.1928, 59.0988) (-60.9926, 59.168) (-60.7931, 59.2365) (-60.5954, 59.303) (-60.4006, 59.3672) (-60.209, 59.4296) (-60.0207, 59.4919) (-59.8349, 59.557) (-59.6507, 59.6284) (-59.4676, 59.7089) (-59.2855, 59.8005) (-59.1052, 59.9038) (-58.9288, 60.0167) (-58.7602, 60.1344) (-58.6052, 60.2482) (-58.47, 60.3489) (-58.3601, 60.4282) (-58.2788, 60.4818) (-58.2263, 60.5108) (-58.1973, 60.5256) (-58.1828, 60.5435) (-58.176, 60.5775) (-58.1802, 60.6236) (-58.2036, 60.667) (-58.2511, 60.694) (-58.3157, 60.7034) (-58.3845, 60.7015) (-58.4433, 60.6972) (-58.4761, 60.696) (-58.4916, 60.6972) (-58.4979, 60.6989) (-58.5, 60.7) knots 0 0 0 0 0 0 0.01052632 0.02105263 0.03157895 0.04210526 0.05263158 0.06315789 0.07368421 0.08421053 0.09473684 0.10526316 0.11578947 0.12631579 0.13684211 0.14736842 0.15789474 0.16842105 0.17894737 0.18947368 0.2 0.21052632 0.22105263 0.23157895 0.24210526 0.25263158 0.26315789 0.27368421 0.28421053 0.29473684 0.30526316 0.31578947 0.32631579 0.33684211 0.34736842 0.35789474 0.36842105 0.37894737 0.38947368 0.4 0.41052632 0.42105263 0.43157895 0.44210526 0.45263158 0.46315789 0.47368421 0.48421053 0.49473684 0.50526316 0.51578947 0.52631579 0.53684211 0.54736842 0.55789474 0.56842105 0.57894737 0.58947368 0.6 0.61052632 0.62105263 0.63157895 0.64210526 0.65263158 0.66315789 0.67368421 0.68421053 0.69473684 0.70526316 0.71578947 0.72631579 0.73684211 0.74736842 0.75789474 0.76842105 0.77894737 0.78947368 0.8 0.81052632 0.82105263 0.83157895 0.84210526 0.85263158 0.86315789 0.87368421 0.88421053 0.89473684 0.90526316 0.91578947 0.92631579 0.93684211 0.94736842 0.95789474 0.96842105 0.97894737 0.98947368 1 1 1 1 1 1
  point P0 (-76.7, 42.3)
  point P1 (-76.0571, 43.4028)
  point P2 (-75.5, 45)
  point P3 (-75.1, 46.8)
  point P4 (-74.9, 48.2)
  point P5 (-74.8, 48.8)
  point P6 (-74.7, 49.15)
  point P7 (-74.3, 49.7)
  point P8 (-73.7, 50.4)
  point P9 (-73.3235, 50.961)
  point P10 (-73.2324, 51.166)
  point P11 (-73.3, 51.3)
  point P12 (-73.7, 51.5)
  point P13 (-74.3, 51.7)
  point P14 (-74.8, 52)
  point P15 (-75.1595, 52.3187)
  point P16 (-75.4, 52.6)
  point P17 (-75.5, 52.9)
  point P18 (-68.7, 59)
  point P19 (-68.4544, 58.7497)
  point P20 (-68.1985, 57.9442)
  point P21 (-67.9, 57.4)
  point P22 (-67.6, 57.1)
  point P23 (-67.1, 57.2)
  point P24 (-66.6, 57.6)
  point P25 (-66.3, 57.9)
  point P26 (-65.6, 58.2)
  point P27 (-64.8, 58.4)
  point P28 (-63.3, 58.6)
  point P29 (-61.8, 58.9)
  point P30 (-60.3, 59.4)
  point P31 (-58.9498, 60.0053)
  point P32 (-58.2486, 60.498)
  point P33 (-58.1822, 60.5549)
  point P34 (-58.2117, 60.6651)
  point P35 (-58.4, 60.7)
  constraint perpendicular L100 L104
  constraint perpendicular L104 L105
  constraint perpendicular L105 L106
  constraint perpendicular L106 L107
  constraint perpendicular L107 L108
  constraint perpendicular L108 L109
  constraint perpendicular L107 L110
  constraint perpendicular L108 L111
  constraint perpendicular L107 L112
  constraint perpendicular L112 L113
  constraint perpendicular L113 L114
  constraint perpendicular L114 L115
  constraint perpendicular L115 L116
  constraint perpendicular L114 L117
  constraint perpendicular L117 L118
  constraint horizontal L119
  constraint vertical L120
  constraint horizontal L121
  constraint vertical L122
  constraint horizontal L123
  constraint vertical L124
  constraint horizontal L125
  constraint vertical L126
  constraint horizontal L127
  constraint vertical L128
  constraint horizontal L129
  constraint vertical L130
  constraint perpendicular L104 L131
  constraint perpendicular L131 L132
  constraint perpendicular L104 L133
  constraint perpendicular L131 L134
  constraint perpendicular L134 L135
  constraint perpendicular L131 L136
  constraint perpendicular L136 L137
  constraint perpendicular L137 L138
  constraint perpendicular L136 L139
  constraint perpendicular L134 L140
  constraint perpendicular L140 L141
extrude "Extrude2" add sketch "Sketch2" along normal blind 0.5 contours L104 L105 L106 L107 L108 L109 L110 L111 L112 L113 L114 L115 L116 L117 L118 L131 L132 L133 L134 L135 L136 L137 L138 L139 L140 L141 S0 S1